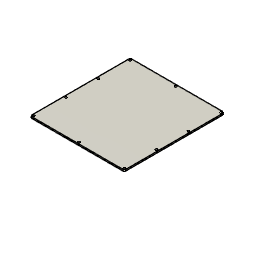
Lid - Pro Compact (Autodesk Fusion 360 design; units mm, degrees)
Autodesk Fusion 360 part; units mm, degrees
note: some values were not read from the file. Set by a fixed rule: which sketch regions a step uses.
sketch "Sketch1" plane through (0, 0, 123.8) normal (0, 0, 1) x (-1, 0, 0)
  line L0 (-99, -172) -> (99, -172)
  arc A0 (99, -172) -> (102, -169) centre (99, -169) ccw
  line L1 (102, -169) -> (102, 41.7937)
  arc A1 (102, 41.7937) -> (99, 44.7937) centre (99, 41.7937) ccw
  line L2 (99, 44.7937) -> (-99, 44.7937)
  arc A2 (-99, 44.7937) -> (-102, 41.7937) centre (-99, 41.7937) ccw
  line L3 (-102, 41.7937) -> (-102, -169)
  arc A3 (-102, -169) -> (-99, -172) centre (-99, -169) ccw
  arc A4 (-94, -154) -> (-84, -164) centre (-84, -154) ccw
  line L4 (-94, -154) -> (-94, 26.7937)
  arc A5 (-84, 36.7937) -> (-94, 26.7937) centre (-84, 26.7937) ccw
  line L5 (-84, 36.7937) -> (84, 36.7937)
  arc A6 (94, 26.7937) -> (84, 36.7937) centre (84, 26.7937) ccw
  line L6 (94, 26.7937) -> (94, -154)
  arc A7 (84, -164) -> (94, -154) centre (84, -154) ccw
  circle A8 centre (-98, -168) radius 1.9
  circle A9 centre (98, -28.804) radius 1.9
  circle A10 centre (-98, 40.7937) radius 1.9
  circle A11 centre (-98, -98.402) radius 1.9
  circle A12 centre (0, 40.7937) radius 1.9
  circle A13 centre (98, -168) radius 1.9
  circle A14 centre (-98, -28.804) radius 1.9
  circle A15 centre (98, 40.7937) radius 1.9
  circle A16 centre (98, -98.402) radius 1.9
  circle A17 centre (0, -168) radius 1.9
  line L7 (-99, -172) -> (-159.6, -172)
  line L8 (84, -164) -> (-84, -164)
  constraint coincident L0.start A3.end
extrude "Extrude1" add sketch "Sketch1" along normal blind 3 contours L0 A0 L1 A1 L2 A2 L3 A3 | A4 L4 A5 L5 A6 L6 A7 L8
sketch "Sketch2" plane through (0, 0, 126.8) normal (0, 0, 1) x (-1, 0, 0)
  circle A0 centre (-98, -98.402) radius 1.9
  circle A1 centre (-98, -168) radius 1.9
  circle A2 centre (98, -98.402) radius 1.9
  circle A3 centre (98, -28.804) radius 1.9
  circle A4 centre (-98, 40.7937) radius 1.9
  circle A5 centre (98, -168) radius 1.9
  circle A6 centre (98, 40.7937) radius 1.9
  circle A7 centre (0, 40.7937) radius 1.9
  circle A8 centre (-98, -28.804) radius 1.9
  circle A9 centre (0, -168) radius 1.9
  arc A10 (99, -172) -> (102, -169) centre (99, -169) ccw
  line L0 (102, -169) -> (102, 41.7937)
  arc A11 (102, 41.7937) -> (99, 44.7937) centre (99, 41.7937) ccw
  line L1 (99, 44.7937) -> (-99, 44.7937)
  arc A12 (-99, 44.7937) -> (-102, 41.7937) centre (-99, 41.7937) ccw
  line L2 (-102, 41.7937) -> (-102, -169)
  arc A13 (-102, -169) -> (-99, -172) centre (-99, -169) ccw
  line L3 (-99, -172) -> (99, -172)
  circle A14 centre (98, -168) radius 2.25
  circle A15 centre (0, -168) radius 2.25
  circle A16 centre (-98, -168) radius 2.25
  circle A17 centre (98, -98.402) radius 2.25
  circle A18 centre (98, -28.804) radius 2.25
  circle A19 centre (-98, -98.402) radius 2.25
  circle A20 centre (-98, -28.804) radius 2.25
  circle A21 centre (98, 40.7937) radius 2.25
  circle A22 centre (0, 40.7937) radius 2.25
  circle A23 centre (-98, 40.7937) radius 2.25
  line L4 (-99, -171.8) -> (99, -171.8)
  arc A24 (99, -171.8) -> (101.8, -169) centre (99, -169) ccw
  line L5 (101.8, -169) -> (101.8, 41.7937)
  arc A25 (101.8, 41.7937) -> (99, 44.5937) centre (99, 41.7937) ccw
  line L6 (99, 44.5937) -> (-99, 44.5937)
  arc A26 (-99, 44.5937) -> (-101.8, 41.7937) centre (-99, 41.7937) ccw
  line L7 (-101.8, 41.7937) -> (-101.8, -169)
  arc A27 (-101.8, -169) -> (-99, -171.8) centre (-99, -169) ccw
  dimension "d1219" = 4.5
  dimension "d1220" = 4.5
  dimension "d1221" = 4.5
  dimension "d1222" = 4.5
  dimension "d1223" = 4.5
  dimension "d1224" = 4.5
  dimension "d1225" = 4.5
  dimension "d1226" = 4.5
  dimension "d1227" = 4.5
  dimension "d1228" = 4.5
  dimension "d1229" = -0.2
  constraint concentric A5 A14
  constraint concentric A9 A15
  constraint concentric A1 A16
  constraint concentric A2 A17
  constraint concentric A3 A18
  constraint concentric A0 A19
  constraint concentric A8 A20
  constraint concentric A6 A21
  constraint concentric A7 A22
  constraint concentric A4 A23
  measures "d1219" diameter of A14
  measures "d1220" diameter of A15
  measures "d1221" diameter of A16
  measures "d1222" diameter of A17
  measures "d1223" diameter of A18
  measures "d1224" diameter of A19
  measures "d1225" diameter of A20
  measures "d1226" diameter of A21
  measures "d1227" diameter of A22
  measures "d1228" diameter of A23
extrude "Extrude2" cut sketch "Sketch2" against normal blind 3
equation "d1220 = d1219"
equation "d1221 = d1219"
equation "d1222 = d1219"
equation "d1223 = d1219"
equation "d1224 = d1219"
equation "d1225 = d1219"
equation "d1226 = d1219"
equation "d1227 = d1219"
equation "d1228 = d1219"
